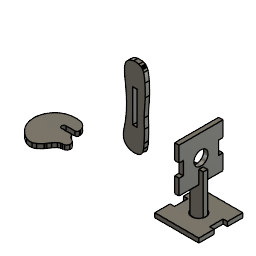
MORFY Test2 (Autodesk Fusion 360 design; units mm, degrees)
Autodesk Fusion 360 part; units mm, degrees
sketch "Sketch1" plane through (0, 0, 0) normal (0, 1, 0) x (1, 0, 0)
  line L0 (0, -100) -> (-100, -100)
  line L1 (-100, -100) -> (-100, 0)
  line L2 (-100, 0) -> (0, 0)
  line L3 (0, 0) -> (0, -100)
  circle A0 centre (-50, -50) radius 16
  line L4 (-130, 0) -> (-160, 0)
  line L5 (-160, 0) -> (-160, -100)
  line L6 (-160, -100) -> (-130, -100)
  line L7 (-130, -100) -> (-130, 0)
  line L8 (-140, -100) -> (-150, -100)
  line L9 (-150, -100) -> (-150, -70)
  line L10 (-150, -70) -> (-140, -70)
  line L11 (-140, -70) -> (-140, -100)
  line L12 (-50, -100) -> (-50, 0) construction
  line L13 (0, -65) -> (-10, -65)
  line L14 (-10, -65) -> (-10, -35)
  line L15 (-10, -35) -> (0, -35)
  line L16 (0, -35) -> (0, -65)
  line L17 (-90, -65) -> (-90, -35)
  line L18 (-100, -65) -> (-90, -65)
  line L19 (-100, -35) -> (-100, -65)
  line L20 (-90, -35) -> (-100, -35)
  line L21 (-190, 0) -> (-290, 0)
  line L22 (-290, 0) -> (-290, -200)
  line L23 (-290, -200) -> (-190, -200)
  line L24 (-190, -200) -> (-190, 0)
  line L25 (-235, -137.5) -> (-245, -137.5)
  line L26 (-245, -137.5) -> (-245, -62.5)
  line L27 (-245, -62.5) -> (-235, -62.5)
  line L28 (-235, -62.5) -> (-235, -137.5)
  line L29 (-240, -200) -> (-240, 0) construction
  line L30 (-235, -100) -> (-245, -100) construction
  line L31 (-320, 0) -> (-450, 0)
  line L32 (-450, 0) -> (-450, -120)
  line L33 (-450, -120) -> (-320, -120)
  line L34 (-320, -120) -> (-320, 0)
  line L35 (-320, -40) -> (-376.3022, -40)
  line L36 (-376.3022, -40) -> (-376.3022, -30)
  line L37 (-376.3022, -30) -> (-320, -30)
  line L38 (-320, -30) -> (-320, -40)
  dimension "d2" = 10
  dimension "d3" = 30
  dimension "d5" = 32
  dimension "d6" = 30
  dimension "d7" = 100
  dimension "d8" = 100
  dimension "d9" = 30
  dimension "d11" = 100
  dimension "d17" = 30
  dimension "d18" = 10
  dimension "d19" = 30
  dimension "d20" = 10
  dimension "d21" = 75
  dimension "d22" = 100
  dimension "d23" = 200
  dimension "d26" = 10
  constraint horizontal L0
  constraint vertical L1
  constraint horizontal L2
  constraint vertical L3
  constraint horizontal L4
  constraint vertical L5
  constraint horizontal L6
  constraint vertical L7
  constraint horizontal L8
  constraint vertical L9
  constraint horizontal L10
  constraint vertical L11
  constraint coincident L6 L8.start
  constraint midpoint L6 L8
  constraint midpoint L0 L12.start
  constraint midpoint L2 L12.end
  constraint midpoint A0.centre L12
  constraint coincident L2.end L3.start
  constraint collinear L2 L4
  constraint horizontal L13
  constraint vertical L14
  constraint horizontal L15
  constraint vertical L16
  constraint collinear L3 L16
  constraint midpoint L3 L16
  constraint symmetric L12 L13.start L18.start
  constraint symmetric L12 L13.end L17.start
  constraint symmetric L12 L14.end L17.end
  constraint symmetric L12 L15.end L19.start
  constraint horizontal L21
  constraint vertical L22
  constraint horizontal L23
  constraint vertical L24
  constraint horizontal L25
  constraint vertical L26
  constraint horizontal L27
  constraint vertical L28
  constraint midpoint L23 L29.start
  constraint midpoint L21 L29.end
  constraint midpoint L28 L30.start
  constraint midpoint L26 L30.end
  constraint midpoint L29 L30
  constraint horizontal L31
  constraint vertical L32
  constraint horizontal L33
  constraint vertical L34
  constraint horizontal L35
  constraint vertical L36
  constraint horizontal L37
  constraint vertical L38
  constraint coincident L34 L35.start
  measures "d2" distance of L9 L11
  measures "d3" distance of L4.start L4.end
  measures "d5" diameter of A0
  measures "d6" distance of L6 L10
  measures "d7" distance of L0.start L0.end
  measures "d8" distance of L0.end L1.end
  measures "d9" distance of L1 L7
  measures "d11" distance of L4.end L5.end
  measures "d17" distance of L13.start L15.end
  measures "d18" distance of L14.end L15.end
  measures "d19" distance of L5 L24
  measures "d20" distance of L25.start L25.end
  measures "d21" distance of L25.end L26.end
  measures "d22" distance of L22.end L23.end
  measures "d23" distance of L21.end L22.end
  measures "d26" distance of L35.start L37.end
extrude "Extrude1" add sketch "Sketch1" along normal blind 10 contours L0 L1 L2 L3 L13 L14 L15 L17 L18 L20 makes body 1
extrude "Extrude2" add sketch "Sketch1" along normal blind 10 separate body contours L4 L5 L6 L7 L9 L10 L11 makes body 2
move_body "Align1" bodies 2 to x (1, 0, 0) y (0, 0, -1) z (0, 1, 0) at (95, 0, 55)
copy_body "CopyPasteBodies1" bodies 1 makes body 3
move_body "Move1" bodies 3 to x (1, 0, 0) y (0, 0, -1) z (0, 1, 0) at (0, 0, 0)
move_body "Align2" bodies 3 to x (0, 0, -1) y (0, 1, 0) z (1, 0, 0) at (-45, 70, 0)
extrude "Extrude3" add sketch "Sketch1" along normal blind 10 separate body contours L21 L22 L23 L24 makes body 4
move_body "Align3" bodies 4 to x (1, 0, 0) y (0, 0, -1) z (0, 1, 0) at (0, 0, 5)
extrude "Extrude4" add sketch "Sketch1" along normal blind 10 separate body contours L31 L32 L33 L34 L35 L36 L37 makes body 5
sketch "Sketch2" plane through (0, 10, 0) normal (0, 1, 0) x (-1, 0, 0)
  line L0 (376.3022, 30) -> (320, 30)
  line L1 (320, 30) -> (320, 0)
  line L2 (320, 0) -> (450, 0)
  line L3 (450, 0) -> (450, 120)
  line L4 (450, 120) -> (320, 120)
  line L5 (320, 120) -> (320, 40)
  line L6 (320, 40) -> (376.3022, 40)
  line L7 (376.3022, 40) -> (376.3022, 30)
  spline S0 degree 3 poles (376.6557, 102.6391) (371.512, 101.3631) (367.0355, 98.0484) (363.3439, 94.3509) knots 0 0 0 0 1 1 1 1
  arc A0 (357.5062, 86.8758) -> (363.3439, 94.3509) centre (391.0598, 66.6885) cw
  arc A1 (357.5062, 86.8758) -> (352.8708, 80.0647) centre (299.0773, 121.6578) cw
  spline S1 degree 3 poles (352.8708, 80.0647) (350.995, 77.6748) (348.9939, 75.2362) (346.5637, 73.3838) knots 0 0 0 0 1 1 1 1
  arc A2 (346.5637, 73.3838) -> (342.1805, 71.337) centre (340.1279, 81.4496) cw
  spline S2 degree 3 poles (342.1805, 71.337) (340.8347, 71.0786) (339.4807, 71.2387) (338.1272, 71.0535) knots 0 0 0 0 1 1 1 1
  arc A3 (333.7152, 69.513) -> (338.1272, 71.0535) centre (339.4277, 60.2412) cw
  arc A4 (328.8829, 62.0589) -> (333.7152, 69.513) centre (339.22, 60.6509) cw
  spline S3 degree 3 poles (328.8829, 62.0589) (328.4961, 58.9796) (329.5175, 55.8298) (331.4461, 53.4285) knots 0 0 0 0 1 1 1 1
  spline S4 degree 3 poles (331.4461, 53.4285) (333.4728, 50.9023) (336.504, 49.5696) (339.247, 47.9992) knots 0 0 0 0 1 1 1 1
  spline S5 degree 3 poles (339.247, 47.9992) (340.6143, 47.2137) (341.9457, 46.3557) (343.032, 45.1963) knots 0 0 0 0 1 1 1 1
  arc A5 (343.032, 45.1963) -> (345.256, 41.0861) centre (336.0059, 38.7378) cw
  spline S6 degree 3 poles (345.256, 41.0861) (346.1709, 37.6717) (345.5238, 34.1527) (345.0459, 30.7335) knots 0 0 0 0 1 1 1 1
  arc A6 (344.6581, 25.2687) -> (345.0459, 30.7335) centre (375.3684, 25.8356) cw
  arc A7 (345.3164, 20.7535) -> (344.6581, 25.2687) centre (366.9426, 26.2119) cw
  arc A8 (356.758, 5.7778) -> (345.3164, 20.7535) centre (368.6021, 26.6855) cw
  spline S7 degree 3 poles (356.758, 5.7778) (362.7758, 2.4342) (369.792, 2.2853) (376.5141, 2.3167) knots 0 0 0 0 1 1 1 1
  arc A9 (390.6655, 4.1292) -> (376.5141, 2.3167) centre (376.6607, 57.3233) cw
  arc A10 (418.8695, 26.6863) -> (390.6655, 4.1292) centre (379.375, 47.1569) cw
  arc A11 (423.7295, 39.7127) -> (418.8695, 26.6863) centre (370.1284, 52.2909) cw
  arc A12 (425.0435, 48.041) -> (423.7295, 39.7127) centre (373.0533, 51.9756) cw
  arc A13 (424.9885, 53.5505) -> (425.0435, 48.041) centre (385.4607, 50.4014) cw
  arc A14 (422.6135, 66.1543) -> (424.9885, 53.5505) centre (369.8994, 49.6952) cw
  arc A15 (414.6238, 81.9198) -> (422.6135, 66.1543) centre (372.037, 50.4304) cw
  arc A16 (408.5747, 88.7752) -> (414.6238, 81.9198) centre (368.1995, 47.0519) cw
  arc A17 (398.0991, 97.2768) -> (408.5747, 88.7752) centre (360.5548, 40.3108) cw
  spline S8 degree 3 poles (398.0991, 97.2768) (393.8305, 100.0641) (389.0443, 102.3299) (383.9447, 102.9869) knots 0 0 0 0 1 1 1 1
  arc A18 (376.6536, 102.6314) -> (383.9447, 102.9869) centre (381.2636, 83.0288) cw
  spline S9 degree 3 poles (376.6536, 102.6314) (375.8256, 102.4342) (376.1738, 101.1576) (377.0025, 101.3574) knots 0 0 0 0 1 1 1 1
  spline S10 degree 3 poles (377.0025, 101.3574) (381.8213, 102.515) (386.8366, 101.4615) (391.2962, 99.4996) knots 0 0 0 0 1 1 1 1
  spline S11 degree 3 poles (391.2962, 99.4996) (395.7558, 97.5377) (399.7961, 94.7267) (403.5, 91.6004) knots 0 0 0 0 1 1 1 1
  arc A19 (403.5, 91.6004) -> (410.6819, 84.6688) centre (356.0679, 35.2687) cw
  arc A20 (410.6819, 84.6688) -> (418.55, 72.8557) centre (373.3041, 51.2467) cw
  arc A21 (418.55, 72.8557) -> (423.0525, 58.6026) centre (370.3385, 49.7882) cw
  arc A22 (423.0525, 58.6026) -> (423.7774, 49.6951) centre (374.0376, 50.1304) cw
  spline S12 degree 3 poles (423.7774, 49.6951) (423.7697, 49.1246) (423.7474, 48.5609) (423.7096, 47.9903) knots 0 0 0 0 1 1 1 1
  spline S13 degree 3 poles (423.7096, 47.9903) (423.6775, 47.5332) (423.6345, 47.0764) (423.5883, 46.6176) knots 0 0 0 0 1 1 1 1
  spline S14 degree 3 poles (423.5883, 46.6176) (423.515, 45.9251) (423.4677, 45.5543) (423.372, 44.9006) knots 0 0 0 0 1 1 1 1
  arc A23 (423.372, 44.9006) -> (420.6414, 33.9634) centre (367.6494, 53.0032) cw
  arc A24 (420.6414, 33.9634) -> (413.3804, 20.5943) centre (374.786, 50.2117) cw
  arc A25 (413.3804, 20.5943) -> (399.1053, 8.7923) centre (379.6025, 46.9163) cw
  arc A26 (399.1053, 8.7923) -> (382.2455, 3.9255) centre (377.7999, 50.9625) cw
  spline S15 degree 3 poles (382.2455, 3.9255) (380.3033, 3.731) (378.3496, 3.6464) (376.3952, 3.6414) knots 0 0 0 0 1 1 1 1
  spline S16 degree 3 poles (376.3952, 3.6414) (373.3248, 3.6424) (370.2289, 3.6502) (367.1779, 3.9993) knots 0 0 0 0 1 1 1 1
  spline S17 degree 3 poles (367.1779, 3.9993) (363.6368, 4.4003) (360.1406, 5.3371) (357.0467, 7.1412) knots 0 0 0 0 1 1 1 1
  arc A27 (357.0467, 7.1412) -> (349.9077, 13.8038) centre (368.2855, 26.3397) cw
  arc A28 (349.9077, 13.8038) -> (346.392, 22.0074) centre (368.6705, 26.7001) cw
  spline S18 degree 3 poles (346.392, 22.0074) (345.686, 25.4041) (346.0944, 28.7378) (346.581, 32.1383) knots 0 0 0 0 1 1 1 1
  spline S19 degree 3 poles (346.581, 32.1383) (347.0453, 35.4351) (347.412, 38.8484) (346.3439, 42.0792) knots 0 0 0 0 1 1 1 1
  arc A29 (343.9732, 46.1329) -> (346.3439, 42.0792) centre (336.0538, 38.7815) cw
  arc A30 (340.3078, 48.912) -> (343.9732, 46.1329) centre (332.347, 34.6053) cw
  spline S20 degree 3 poles (340.3078, 48.912) (337.6368, 50.485) (334.6236, 51.7115) (332.5733, 54.129) knots 0 0 0 0 1 1 1 1
  spline S21 degree 3 poles (332.5733, 54.129) (330.676, 56.3713) (329.7148, 59.5515) (330.2751, 62.4501) knots 0 0 0 0 1 1 1 1
  arc A31 (330.2751, 62.4501) -> (335.5719, 69.01) centre (339.3201, 60.5652) cw
  arc A32 (335.5719, 69.01) -> (339.6905, 69.8238) centre (339.5084, 59.9169) cw
  arc A33 (343.2167, 70.2157) -> (339.6905, 69.8238) centre (339.9467, 83.5798) cw
  spline S22 degree 3 poles (343.2167, 70.2157) (344.9644, 70.676) (346.5059, 71.6243) (347.8953, 72.7613) knots 0 0 0 0 1 1 1 1
  spline S23 degree 3 poles (347.8953, 72.7613) (350.3244, 74.7428) (352.3351, 77.2171) (354.2448, 79.6829) knots 0 0 0 0 1 1 1 1
  arc A34 (358.6744, 86.2368) -> (354.2448, 79.6829) centre (298.1579, 122.3635) cw
  spline S24 degree 3 poles (358.6744, 86.2368) (359.2158, 87.1327) (359.7685, 88.02) (360.3701, 88.875) knots 0 0 0 0 1 1 1 1
  spline S25 degree 3 poles (360.3701, 88.875) (360.5357, 89.1045) (360.7013, 89.3341) (360.8787, 89.5769) knots 0 0 0 0 1 1 1 1
  line L8 (360.8787, 89.5769) -> (361.0093, 89.7474)
  spline S26 degree 3 poles (361.0093, 89.7474) (360.8905, 89.5902) (361.0663, 89.817) (361.1214, 89.8899) knots 0 0 0 0 1 1 1 1
  arc A35 (361.1214, 89.8899) -> (369.8963, 98.1036) centre (391.8914, 65.8119) cw
  arc A36 (369.8963, 98.1036) -> (376.9943, 101.3678) centre (382.8335, 79.3209) cw
  spline S27 degree 3 poles (376.9943, 101.3678) (377.8314, 101.5681) (377.4832, 102.8447) (376.6557, 102.6391) knots 0 0 0 0 1 1 1 1
extrude "Extrude5" cut sketch "Sketch2" against normal up to surface (10 mm away) contours L0 L6 L7 S9 S10 S11 A19 A20 A21 A22 S12 S13 S14 A23 A24 A25 A26 S15 S16 S17 A27 A28 S18 S19 A29 A30 S20 S21 A31 A32 A33 S22 S23 A34 S24 S25 L8 S26 A35 A36 keep common part bodies 5
fillet "Fillet1" radius 5 4 edges at (-346.2939, 5, 30) (-346.8429, 5, 40) (-376.3022, 5, 30) (-376.3022, 5, 40) on bodies 5
sketch "Sketch3" plane through (0, 0, -5) normal (0, 0, -1) x (-1, 0, 0)
  line L0 (245, 62.5) -> (235, 62.5)
  line L1 (235, 62.5) -> (235, 137.5)
  line L2 (235, 137.5) -> (245, 137.5)
  line L3 (245, 137.5) -> (245, 62.5)
  line L4 (190, 200) -> (190, 0)
  line L5 (190, 0) -> (290, 0)
  line L6 (290, 0) -> (290, 200)
  line L7 (290, 200) -> (190, 200)
  arc A0 (231.0803, 191.0905) -> (255.6552, 187.0617) centre (238.751, 160.9144) cw
  spline S0 degree 3 poles (231.0803, 191.0905) (226.8847, 189.9814) (222.8559, 187.783) (220.4416, 184.0831) knots 0 0 0 0 1 1 1 1
  spline S1 degree 3 poles (220.4416, 184.0831) (218.0273, 180.3831) (217.0753, 175.7949) (216.3491, 171.5159) knots 0 0 0 0 1 1 1 1
  spline S2 degree 3 poles (216.3491, 171.5159) (214.8426, 162.5997) (214.4157, 153.4773) (214.1605, 144.4531) knots 0 0 0 0 1 1 1 1
  spline S3 degree 3 poles (214.1605, 144.4531) (213.9249, 136.1601) (214.0623, 127.867) (214.6512, 119.5887) knots 0 0 0 0 1 1 1 1
  spline S4 degree 3 poles (214.6512, 119.5887) (215.1125, 113.0916) (215.8142, 106.6093) (216.2166, 100.1025) knots 0 0 0 0 1 1 1 1
  arc A1 (216.2166, 100.1025) -> (216.3393, 75.2528) centre (-14.0194, 86.5407) cw
  spline S5 degree 3 poles (216.3393, 75.2528) (216.0007, 67.8626) (215.7553, 60.4872) (215.981, 53.0824) knots 0 0 0 0 1 1 1 1
  spline S6 degree 3 poles (215.981, 53.0824) (216.1381, 47.8465) (216.4717, 42.6155) (216.8643, 37.3796) knots 0 0 0 0 1 1 1 1
  spline S7 degree 3 poles (216.8643, 37.3796) (217.1538, 33.4539) (217.4875, 29.5576) (218.1549, 25.6957) knots 0 0 0 0 1 1 1 1
  spline S8 degree 3 poles (218.1549, 25.6957) (219.0971, 20.234) (220.9176, 14.9344) (225.4861, 11.465) knots 0 0 0 0 1 1 1 1
  spline S9 degree 3 poles (225.4861, 11.465) (231.3747, 7.0486) (239.3831, 6.1751) (246.469, 7.2792) knots 0 0 0 0 1 1 1 1
  spline S10 degree 3 poles (246.469, 7.2792) (253.7561, 8.4128) (261.1904, 11.995) (265.2143, 18.3792) knots 0 0 0 0 1 1 1 1
  spline S11 degree 3 poles (265.2143, 18.3792) (269.7779, 25.573) (269.1939, 34.6708) (267.8837, 42.7185) knots 0 0 0 0 1 1 1 1
  spline S12 degree 3 poles (267.8837, 42.7185) (267.1967, 46.9632) (266.2349, 51.1588) (265.4302, 55.3838) knots 0 0 0 0 1 1 1 1
  spline S13 degree 2 poles (265.4302, 55.3838) (264.0415, 62.9163) (263.1533, 70.5223) knots 0 0 0 1 1 1
  spline S14 degree 3 poles (263.1533, 70.5223) (261.1904, 87.6973) (261.2787, 104.9949) (262.7558, 122.1993) knots 0 0 0 0 1 1 1 1
  spline S15 degree 3 poles (262.7558, 122.1993) (263.3397, 128.976) (264.12, 135.7381) (264.8659, 142.5001) knots 0 0 0 0 1 1 1 1
  spline S16 degree 3 poles (264.8659, 142.5001) (265.4793, 148.0697) (266.0877, 153.654) (266.2742, 159.2579) knots 0 0 0 0 1 1 1 1
  spline S17 degree 3 poles (266.2742, 159.2579) (266.5441, 167.5706) (265.862, 176.6635) (260.101, 183.1802) knots 0 0 0 0 1 1 1 1
  arc A2 (255.6306, 187.0323) -> (260.101, 183.1802) centre (242.9117, 167.7518) cw
  spline S18 degree 3 poles (255.6306, 187.0323) (254.3155, 187.9156) (253.0887, 185.7908) (254.394, 184.9124) knots 0 0 0 0 1 1 1 1
  arc A3 (254.394, 184.9124) -> (258.5896, 181.1879) centre (243.0847, 167.9473) cw
  spline S19 degree 3 poles (258.5896, 181.1879) (258.9184, 180.8051) (259.0362, 180.6579) (259.2423, 180.3782) knots 0 0 0 0 1 1 1 1
  spline S20 degree 3 poles (259.2423, 180.3782) (259.5318, 179.9856) (259.8115, 179.5832) (260.0716, 179.171) knots 0 0 0 0 1 1 1 1
  arc A4 (260.0716, 179.171) -> (261.3573, 176.8009) centre (242.7796, 168.2574) cw
  arc A5 (261.3573, 176.8009) -> (261.8136, 175.7312) centre (251.0598, 171.7758) cw
  spline S21 degree 3 poles (261.8136, 175.7312) (261.9805, 175.2993) (262.1326, 174.8626) (262.2749, 174.4209) knots 0 0 0 0 1 1 1 1
  arc A6 (262.2749, 174.4209) -> (263.011, 171.6582) centre (235.3513, 165.7683) cw
  arc A7 (263.011, 171.6582) -> (263.7765, 165.593) centre (227.5288, 164.099) cw
  arc A8 (263.7765, 165.593) -> (263.2858, 150.8716) centre (160.9642, 161.6512) cw
  spline S22 degree 3 poles (263.2858, 150.8716) (262.7411, 144.7966) (261.9952, 138.7412) (261.3229, 132.676) knots 0 0 0 0 1 1 1 1
  spline S23 degree 3 poles (261.3229, 132.676) (259.6643, 117.1989) (258.6927, 101.663) (259.4288, 86.0975) knots 0 0 0 0 1 1 1 1
  arc A9 (262.6037, 57.2534) -> (259.4288, 86.0975) centre (493.4438, 97.2591) cw
  spline S24 degree 3 poles (262.6037, 57.2534) (264.0415, 48.9702) (266.4361, 40.6821) (266.3331, 32.2271) knots 0 0 0 0 1 1 1 1
  spline S25 degree 3 poles (266.3331, 32.2271) (266.2889, 28.3357) (265.6559, 24.3757) (263.8108, 20.8965) knots 0 0 0 0 1 1 1 1
  arc A10 (263.8108, 20.8965) -> (256.4501, 13.3739) centre (246.7128, 30.2641) cw
  arc A11 (256.4501, 13.3739) -> (235.6439, 9.7721) centre (241.1897, 39.6316) cw
  spline S26 degree 3 poles (235.6439, 9.7721) (230.0007, 10.8516) (224.8482, 13.7419) (222.4781, 19.0514) knots 0 0 0 0 1 1 1 1
  spline S27 degree 3 poles (222.4781, 19.0514) (221.3249, 21.6326) (220.7459, 24.5425) (220.3091, 27.3445) knots 0 0 0 0 1 1 1 1
  spline S28 degree 3 poles (220.3091, 27.3445) (219.7105, 31.2162) (219.4258, 35.1419) (219.1559, 39.0529) knots 0 0 0 0 1 1 1 1
  spline S29 degree 3 poles (219.1559, 39.0529) (218.5082, 48.3764) (218.1107, 57.7) (218.3953, 67.0579) knots 0 0 0 0 1 1 1 1
  spline S30 degree 3 poles (218.3953, 67.0579) (218.6211, 74.4186) (219.0971, 81.7498) (219.0235, 89.1154) knots 0 0 0 0 1 1 1 1
  spline S31 degree 3 poles (219.0235, 89.1154) (218.8861, 102.718) (216.9281, 116.2028) (216.5699, 129.7906) knots 0 0 0 0 1 1 1 1
  arc A12 (216.5699, 129.7906) -> (217.2765, 158.1784) centre (497.4595, 137.0014) cw
  spline S32 degree 3 poles (217.2765, 158.1784) (217.7672, 164.6754) (218.3168, 171.3687) (220.2208, 177.6253) knots 0 0 0 0 1 1 1 1
  arc A13 (220.2208, 177.6253) -> (222.2376, 182.3558) centre (238.6742, 172.5529) cw
  spline S33 degree 3 poles (222.2376, 182.3558) (222.4192, 182.66) (222.6106, 182.9594) (222.8167, 183.2489) knots 0 0 0 0 1 1 1 1
  spline S34 degree 3 poles (222.8167, 183.2489) (222.9099, 183.3863) (223.0129, 183.5188) (223.1111, 183.6513) knots 0 0 0 0 1 1 1 1
  spline S35 degree 3 poles (223.1111, 183.6513) (222.8952, 183.3667) (223.2141, 183.774) (223.273, 183.8427) knots 0 0 0 0 1 1 1 1
  arc A14 (223.273, 183.8427) -> (224.5587, 185.1578) centre (232.8394, 175.7764) cw
  line L8 (224.5587, 185.1578) -> (224.8629, 185.4129)
  spline S36 degree 3 poles (224.8629, 185.4129) (224.9365, 185.4718) (225.3242, 185.7712) (225.0003, 185.5258) knots 0 0 0 0 1 1 1 1
  spline S37 degree 3 poles (225.0003, 185.5258) (225.4027, 185.83) (225.8149, 186.1196) (226.2467, 186.3895) knots 0 0 0 0 1 1 1 1
  arc A15 (226.2467, 186.3895) -> (231.2324, 188.5682) centre (236.4245, 169.8934) cw
  arc A16 (231.2324, 188.5682) -> (243.1224, 189.2405) centre (238.7045, 161.8943) cw
  arc A17 (243.1224, 189.2405) -> (254.4088, 184.9516) centre (238.8856, 161.0962) cw
  spline S38 degree 3 poles (254.4088, 184.9516) (255.7386, 184.0684) (256.9654, 186.1931) (255.6552, 187.0617) knots 0 0 0 0 1 1 1 1
extrude "Extrude6" cut sketch "Sketch3" against normal up to surface (10 mm away) contours S18 A3 S19 S20 A4 A5 S21 A6 A7 A8 S22 S23 A9 S24 S25 A10 A11 S26 S27 S28 S29 S30 S31 A12 S32 A13 S33 S34 S35 A14 L8 S36 S37 A15 A16 A17 keep common part bodies 4
equation "espressura = 10 mm"
equation "d2 = espressura"
equation "d3 = diameter"
equation "diameter = 30 mm"
equation "d5 = diameter + plus"
equation "d6 = diameter"
equation "d8 = d7"
equation "d9 = distance"
equation "distance = 30 mm"
equation "d11 = d7"
equation "d12 = espressura"
equation "d14 = espressura"
equation "plus = 2 mm"
equation "d17 = diameter"
equation "d18 = espressura"
equation "d19 = distance"
equation "d20 = espressura"
equation "d21 = d11 - ( d11 / 4 )"
equation "d24 = espressura"
equation "d26 = espressura"
equation "d27 = espressura"
